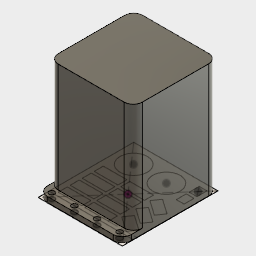
size_test (Autodesk Fusion 360 design; units mm, degrees)
Autodesk Fusion 360 part; units mm, degrees
sketch "Sketch1" plane through (0, 0, 0) normal (0, 1, 0) x (1, 0, 0)
  line L0 (23.1297, 26.25) -> (-23.1297, 26.25)
  line L1 (-23.1297, 26.25) -> (-23.1297, -26.25)
  line L2 (-23.1297, -26.25) -> (23.1297, -26.25)
  line L3 (23.1297, -26.25) -> (23.1297, 26.25)
  line L4 (23.1297, 26.25) -> (-23.1297, -26.25) construction
  line L5 (-23.1297, 26.25) -> (23.1297, -26.25) construction
  line L6 (-20.1297, -18.25) -> (-7.1297, -18.25)
  line L7 (-7.1297, -18.25) -> (-7.1297, -13.25)
  line L8 (-7.1297, -13.25) -> (-20.1297, -13.25)
  line L9 (-20.1297, -13.25) -> (-20.1297, -18.25)
  circle A0 centre (-12.6297, 15.75) radius 7.5
  line L10 (-5.5297, -13.25) -> (-5.5297, -18.25)
  line L11 (7.4703, -13.25) -> (-5.5297, -13.25)
  line L12 (7.4703, -18.25) -> (7.4703, -13.25)
  line L13 (-5.5297, -18.25) -> (7.4703, -18.25)
  line L14 (-20.1297, -6.65) -> (-20.1297, -11.65)
  line L15 (-7.1297, -6.65) -> (-20.1297, -6.65)
  line L16 (-7.1297, -11.65) -> (-7.1297, -6.65)
  line L17 (-20.1297, -11.65) -> (-7.1297, -11.65)
  line L18 (-5.5297, -6.65) -> (-5.5297, -11.65)
  line L19 (7.4703, -6.65) -> (-5.5297, -6.65)
  line L20 (7.4703, -11.65) -> (7.4703, -6.65)
  line L21 (-5.5297, -11.65) -> (7.4703, -11.65)
  line L22 (-20.1297, -0.05) -> (-20.1297, -5.05)
  line L23 (-7.1297, -0.05) -> (-20.1297, -0.05)
  line L24 (-7.1297, -5.05) -> (-7.1297, -0.05)
  line L25 (-20.1297, -5.05) -> (-7.1297, -5.05)
  line L26 (-5.5297, -0.05) -> (-5.5297, -5.05)
  line L27 (7.4703, -0.05) -> (-5.5297, -0.05)
  line L28 (7.4703, -5.05) -> (7.4703, -0.05)
  line L29 (-5.5297, -5.05) -> (7.4703, -5.05)
  line L30 (-20.1297, 6.55) -> (-20.1297, 1.55)
  line L31 (-7.1297, 6.55) -> (-20.1297, 6.55)
  line L32 (-7.1297, 1.55) -> (-7.1297, 6.55)
  line L33 (-20.1297, 1.55) -> (-7.1297, 1.55)
  line L34 (-5.5297, 6.55) -> (-5.5297, 1.55)
  line L35 (7.4703, 6.55) -> (-5.5297, 6.55)
  line L36 (7.4703, 1.55) -> (7.4703, 6.55)
  line L37 (-5.5297, 1.55) -> (7.4703, 1.55)
  line L38 (7.4703, -18.25) -> (23.1297, -18.25) construction
  line L39 (17.2618, -18.25) -> (9.0703, -12.5142)
  line L40 (9.0703, -12.5142) -> (11.9382, -8.4185)
  line L41 (11.9382, -8.4185) -> (20.1297, -14.1542)
  line L42 (20.1297, -14.1542) -> (17.2618, -18.25)
  line L43 (17.2618, -10.514) -> (9.0703, -4.7782)
  line L44 (9.0703, -4.7782) -> (11.9382, -0.6825)
  line L45 (11.9382, -0.6825) -> (20.1297, -6.4182)
  line L46 (20.1297, -6.4182) -> (17.2618, -10.514)
  line L47 (17.2618, -2.778) -> (9.0703, 2.9578)
  line L48 (9.0703, 2.9578) -> (11.9382, 7.0535)
  line L49 (11.9382, 7.0535) -> (20.1297, 1.3178)
  line L50 (20.1297, 1.3178) -> (17.2618, -2.778)
  circle A1 centre (5.3703, 15.75) radius 7.5
  line L51 (20.1297, 23.25) -> (15.8797, 23.25)
  line L52 (15.8797, 23.25) -> (15.8797, 17.75)
  line L53 (15.8797, 17.75) -> (20.1297, 17.75)
  line L54 (20.1297, 17.75) -> (20.1297, 23.25)
  line L55 (20.1297, 23.25) -> (15.8797, 17.75) construction
  line L56 (15.8797, 23.25) -> (20.1297, 17.75) construction
  line L57 (20.1297, 10.65) -> (20.1297, 16.15)
  line L58 (15.8797, 16.15) -> (15.8797, 10.65)
  line L59 (15.8797, 10.65) -> (20.1297, 10.65)
  line L60 (20.1297, 16.15) -> (15.8797, 16.15)
  circle A2 centre (-18.6297, -23.25) radius 1.5
  line L61 (-23.1297, -20.25) -> (23.1297, -20.25)
  circle A3 centre (-6.2104, -23.25) radius 1.5
  circle A4 centre (6.209, -23.25) radius 1.5
  circle A5 centre (18.6283, -23.25) radius 1.5
  point P0 (18.0047, 20.5)
  dimension "d1" = 13
  dimension "d2" = 5
  dimension "d4" = 3
  dimension "d5" = 15
  dimension "d6" = 10.5
  dimension "d7" = 10.5
  dimension "d8" = 52.5
  dimension "d11" = 14.6
  dimension "d12" = 6.6
  dimension "d16" = 35
  dimension "d17" = 1.6
  dimension "d18" = 10
  dimension "d19" = 5
  dimension "d21" = 3
  dimension "d24" = 0
  dimension "d25" = 7.736
  dimension "d28" = 18
  dimension "d29" = 0
  dimension "d36" = 4.25
  dimension "d37" = 5.5
  dimension "d38" = 3
  dimension "d39" = 3
  dimension "d42" = 0
  dimension "d43" = -7.1
  dimension "d44" = 3
  dimension "d46" = 4.5
  dimension "d47" = 3
  dimension "d48" = 6
  dimension "d49" = 2
  dimension "d52" = 37.258
  dimension "d53" = 0
  measures "d1" distance of L6.start L6.end
  measures "d2" distance of L6.end L7.end
  measures "d4" distance of L1 L9
  measures "d5" diameter of A0
  measures "d6" distance of L0 A0.centre
  measures "d7" distance of L1 A0.centre
  measures "d8" distance of L0.end L1.end
  measures "d16" angle of L38 L39
  measures "d17" distance of L12 L39.end
  measures "d18" distance of L39.start L39.end
  measures "d19" distance of L39.end L40.end
  measures "d21" distance of L3 L41.end
  measures "d36" distance of L51.start L52.end
  measures "d37" distance of L51.start L53.end
  measures "d38" distance of L3 L54
  measures "d39" distance of L0 L51
  measures "d44" diameter of A2
  measures "d46" distance of L1 A2.centre
  measures "d47" distance of L2 A2.centre
  measures "d48" distance of L2 L61
  measures "d49" distance of L6 L61
extrude "Extrude3" add sketch "Sketch1" along normal blind 3
extrude "Extrude4" add sketch "Sketch1" along normal blind 58 from surface at 3 contours L0 L1 L3 L61
extrude "Extrude5" add sketch "Sketch1" along normal blind 2 from surface at 61 contours L0 L1 L3 L61 | L6 L7 L8 L9 | A0 | L10 L11 L12 L13 | L14 L15 L16 L17 | L18 L19 L20 L21 | L22 L23 L24 L25 | L26 L27 L28 L29 | L30 L31 L32 L33 | L34 L35 L36 L37 | L39 L40 L41 L42 | L43 L44 L45 L46 | L47 L48 L49 L50 | A1 | L51 L52 L53 L54 | L57 L58 L59 L60
fillet "Fillet2" radius 5 6 edges at (23.1297, 1.5, 26.25) (23.1297, 33, 20.25) (-23.1297, 1.5, 26.25) (-23.1297, 33, 20.25) (23.1297, 31.5, -26.25) (-23.1297, 31.5, -26.25)
equation "d6 = 7.5 mm + 3 mm"
equation "d25 = 5.736 mm + 2 mm"
equation "d43 = -5.5 mm - 1.6 mm"
